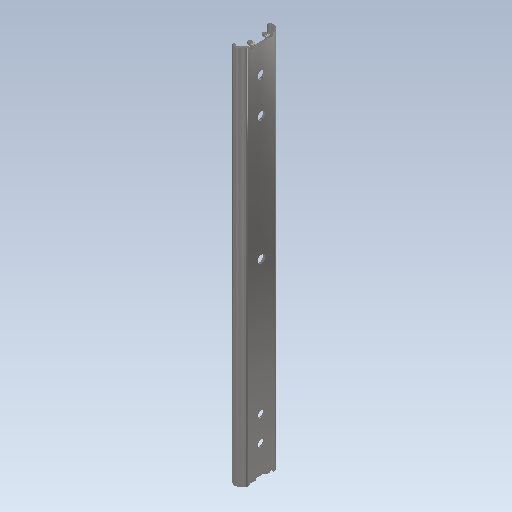
# Autodesk Inventor part: SSRC215_or
Saved by Autodesk Inventor 2021.2 (Build 252289000, 289)
## iProperties
Part Number: SSRC215_or
Material: ステンレス鋼
Catalog Web Link: www.cadenas.de
Description: SSRC2_outer_rail-Slide Rails - Load Rating: 137N ~ 177N/2 pcs - Light Load / Compact - Stainless Steel - Tow-Step
Vendor: MISUMI
Document SubType Name: Modeling
Designer: partserver
Manufacturer: MISUMI
Mass: 19.4626 g
Surface Area: 63.9405 cm^2
Volume: 2.43283 cm^3
Density: 8 g/cm^3
Appearance: 半つや出し
Category: PARTsolutions
Company: MISUMI
PSOL_IDENT_0: {$CADENAS_DATA\23d-libs\misumi\metric\07_slide_rails\ssrc2\ssrc2_outer_rail.prj},167 {VTYP=3D},{NB=S
PSOL_IDENT_1: SRC215_or},{LINA=SSRC215},{NN=SSRC2_outer_rail},{DATE=30.03.2018 01:39:53},{GEOMDATE=30.06.2015 02:0
PSOL_IDENT_2: 1:15},{VERSION=},{LINEID=30},{WBVAR=},{WBNUMERIC=}  {NB=SSRC215_or},{LINA=SSRC215},{KT=DUMMY},{PN=SS
PSOL_IDENT_3: RC215},{TYPE=SSRC2},{NO=15},{L=150},{S=94.5},{A=63},{B=126},{C=63},{D=126},{E=102},{F=98}
NB: SSRC215_or
NN: SSRC2_outer_rail
NT: Slide Rails - Load Rating: 137N ~ 177N/2 pcs - Light Load / Compact - Stainless Steel - Tow-Step
NBSYN: $PN._or
LINA: SSRC215
CATALOG: Misumi
PN: SSRC215
NO: 15
L: 150
S: 94.5
A: 63
B: 126
C: 63
D: 126
E: 102
F: 98
SUPPLIER: MISUMI
ARTICLENO: SSRC215_or
BOMINFO: SSRC215
CREATOR: CADENAS GmbH
Title: SSRC215
Author: Cadenas PARTsolutions
Comments: Slide Rails - Load Rating: 137N ~ 177N/2 pcs - Light Load / Compact - Stainless Steel - Tow-Step
Autodesk Inventor part; units mm, degrees
sketch "_____1" plane through (0, 0, 0) normal (0, 0, 1) x (1, 0, 0)
  line L0 (-2.85, 5.26) -> (-2.85, -5.26)
  arc A0 (-2.85, -5.26) -> (-2.0307, -6.4679) centre (-1.55, -5.26) ccw
  line L1 (-2.0307, -6.4679) -> (-1.8349, -6.5458)
  arc A1 (-1.8349, -6.5458) -> (1.43, -7.1482) centre (0, -5.75) ccw
  line L2 (1.43, -7.1482) -> (1.43, -6.5756)
  line L3 (1.43, -6.5756) -> (1.0392, -6.35)
  arc A2 (-1.1009, -6.2275) -> (1.0392, -6.35) centre (0, -5.75) ccw
  arc A3 (-1.1009, -6.2275) -> (-1.5391, -5.8025) centre (-1.8349, -6.5458) ccw
  line L4 (-1.5391, -5.8025) -> (-1.7349, -5.7246)
  arc A4 (-2.05, -5.26) -> (-1.7349, -5.7246) centre (-1.55, -5.26) ccw
  line L5 (-2.05, -5.26) -> (-2.05, 5.26)
  arc A5 (-1.7349, 5.7246) -> (-2.05, 5.26) centre (-1.55, 5.26) ccw
  line L6 (-1.7349, 5.7246) -> (-1.5391, 5.8025)
  arc A6 (-1.5391, 5.8025) -> (-1.1009, 6.2275) centre (-1.8349, 6.5458) ccw
  arc A7 (1.0392, 6.35) -> (-1.1009, 6.2275) centre (0, 5.75) ccw
  line L7 (1.0392, 6.35) -> (1.43, 6.5756)
  line L8 (1.43, 6.5756) -> (1.43, 7.1482)
  arc A8 (1.43, 7.1482) -> (-1.8349, 6.5458) centre (0, 5.75) ccw
  line L9 (-1.8349, 6.5458) -> (-2.0307, 6.4679)
  arc A9 (-2.0307, 6.4679) -> (-2.85, 5.26) centre (-1.55, 5.26) ccw
  constraints: 20 end point, 20 point on circle, 10 centre point
extrude "Extrusion1" add sketch "_____1" against normal blind 150
sketch "_____3" plane through (0, 0, 0) normal (0, 0, 1) x (1, 0, 0)
  line L0 (-2.05, 3.6) -> (-2.05, 2.2)
  line L1 (-2.05, 2.2) -> (-0.95, 2.2)
  arc A0 (-0.95, 2.2) -> (-0.45, 2.7) centre (-0.95, 2.7) ccw
  line L2 (-0.45, 2.7) -> (-0.45, 2.9484)
  arc A1 (-0.45, 2.9484) -> (-0.8206, 3.4314) centre (-0.95, 2.9484) ccw
  line L3 (-0.8206, 3.4314) -> (-1.45, 3.6)
  line L4 (-1.45, 3.6) -> (-2.05, 3.6)
  constraints: 10 end point, 4 point on circle, 2 centre point
extrude "Extrusion2" add sketch "_____3" against normal blind 0.8
sketch "_____5" plane through (0, 0, 0) normal (0, 0, 1) x (1, 0, 0)
  line L0 (-2.05, -3.6) -> (-1.45, -3.6)
  line L1 (-1.45, -3.6) -> (-0.8206, -3.4314)
  arc A0 (-0.8206, -3.4314) -> (-0.45, -2.9484) centre (-0.95, -2.9484) ccw
  line L2 (-0.45, -2.9484) -> (-0.45, -2.7)
  arc A1 (-0.45, -2.7) -> (-0.95, -2.2) centre (-0.95, -2.7) ccw
  line L3 (-0.95, -2.2) -> (-2.05, -2.2)
  line L4 (-2.05, -2.2) -> (-2.05, -3.6)
  constraints: 10 end point, 4 point on circle, 2 centre point
extrude "Extrusion3" add sketch "_____5" against normal blind 0.8
sketch "_____4" plane through (0, 0, 0) normal (1, 0, 0) x (0, 1, 0)
  line L0 (7.75, 1) -> (-7.75, 1)
  line L1 (-7.75, 1) -> (-7.75, 0)
  line L2 (-7.75, 0) -> (-4.9, 0)
  arc A0 (-4.6, -0.3) -> (-4.9, 0) centre (-4.9, -0.3) ccw
  line L3 (-4.6, -0.3) -> (-4.6, -0.7)
  arc A1 (-4.6, -0.7) -> (-4.1, -1.2) centre (-4.1, -0.7) ccw
  arc A2 (-4.1, -1.2) -> (-3.6, -0.7) centre (-4.1, -0.7) ccw
  line L4 (-3.6, -0.7) -> (-3.6, 0)
  line L5 (-3.6, 0) -> (-2.2, 0)
  line L6 (-2.2, 0) -> (-2.2, -0.7)
  arc A3 (-2.2, -0.7) -> (-1.7, -1.2) centre (-1.7, -0.7) ccw
  line L7 (-1.7, -1.2) -> (1.7, -1.2)
  arc A4 (1.7, -1.2) -> (2.2, -0.7) centre (1.7, -0.7) ccw
  line L8 (2.2, -0.7) -> (2.2, 0)
  line L9 (2.2, 0) -> (3.6, 0)
  line L10 (3.6, 0) -> (3.6, -0.7)
  arc A5 (3.6, -0.7) -> (4.1, -1.2) centre (4.1, -0.7) ccw
  arc A6 (4.1, -1.2) -> (4.6, -0.7) centre (4.1, -0.7) ccw
  line L11 (4.6, -0.7) -> (4.6, -0.3)
  arc A7 (4.9, 0) -> (4.6, -0.3) centre (4.9, -0.3) ccw
  line L12 (4.9, 0) -> (7.75, 0)
  line L13 (7.75, 0) -> (7.75, 1)
  constraints: 28 end point, 16 point on circle, 8 centre point
extrude "Extrusion4" cut sketch "_____4" against normal blind 4.28
sketch "_____6" plane through (0, 0, 0) normal (0, 1, 0) x (1, 0, 0)
  line L0 (-2.85, 0.8) -> (-2.85, 0)
  line L1 (-2.85, 0) -> (-2.05, 0)
  arc A0 (-2.85, 0.8) -> (-2.05, 0) centre (-2.05, 0.8) ccw
  constraints: 4 end point, 2 point on circle, 1 centre point
extrude "Extrusion5" cut sketch "_____6" along normal mid plane 8.2
sketch "_____2" plane through (0, 0, -150) normal (0, 0, 1) x (1, 0, 0)
  line L0 (-2.05, 3.6) -> (-2.05, 2.2)
  line L1 (-2.05, 2.2) -> (-0.95, 2.2)
  arc A0 (-0.95, 2.2) -> (-0.45, 2.7) centre (-0.95, 2.7) ccw
  line L2 (-0.45, 2.7) -> (-0.45, 2.9484)
  arc A1 (-0.45, 2.9484) -> (-0.8206, 3.4314) centre (-0.95, 2.9484) ccw
  line L3 (-0.8206, 3.4314) -> (-1.45, 3.6)
  line L4 (-1.45, 3.6) -> (-2.05, 3.6)
  constraints: 10 end point, 4 point on circle, 2 centre point
extrude "Extrusion6" add sketch "_____2" along normal blind 0.8
sketch "_____7" plane through (0, 0, -150) normal (0, 0, 1) x (1, 0, 0)
  line L0 (-2.05, -3.6) -> (-1.45, -3.6)
  line L1 (-1.45, -3.6) -> (-0.8206, -3.4314)
  arc A0 (-0.8206, -3.4314) -> (-0.45, -2.9484) centre (-0.95, -2.9484) ccw
  line L2 (-0.45, -2.9484) -> (-0.45, -2.7)
  arc A1 (-0.45, -2.7) -> (-0.95, -2.2) centre (-0.95, -2.7) ccw
  line L3 (-0.95, -2.2) -> (-2.05, -2.2)
  line L4 (-2.05, -2.2) -> (-2.05, -3.6)
  constraints: 10 end point, 4 point on circle, 2 centre point
extrude "Extrusion7" add sketch "_____7" along normal blind 0.8
sketch "_____8" plane through (-2.85, 0, 0) normal (1, 0, 0) x (0, 0, -1)
  arc A0 (148.8, -4.1) -> (149.3, -4.6) centre (149.3, -4.1) ccw
  line L0 (149.3, -4.6) -> (149.7, -4.6)
  arc A1 (150, -4.9) -> (149.7, -4.6) centre (149.7, -4.9) ccw
  line L1 (150, -4.9) -> (150, -7.75)
  line L2 (150, -7.75) -> (151, -7.75)
  line L3 (151, -7.75) -> (151, 7.75)
  line L4 (151, 7.75) -> (150, 7.75)
  line L5 (150, 7.75) -> (150, 4.9)
  arc A2 (149.7, 4.6) -> (150, 4.9) centre (149.7, 4.9) ccw
  line L6 (149.7, 4.6) -> (149.3, 4.6)
  arc A3 (149.3, 4.6) -> (148.8, 4.1) centre (149.3, 4.1) ccw
  arc A4 (148.8, 4.1) -> (149.3, 3.6) centre (149.3, 4.1) ccw
  line L7 (149.3, 3.6) -> (150, 3.6)
  line L8 (150, 3.6) -> (150, 2.2)
  line L9 (150, 2.2) -> (149.3, 2.2)
  arc A5 (149.3, 2.2) -> (148.8, 1.7) centre (149.3, 1.7) ccw
  line L10 (148.8, 1.7) -> (148.8, -1.7)
  arc A6 (148.8, -1.7) -> (149.3, -2.2) centre (149.3, -1.7) ccw
  line L11 (149.3, -2.2) -> (150, -2.2)
  line L12 (150, -2.2) -> (150, -3.6)
  line L13 (150, -3.6) -> (149.3, -3.6)
  arc A7 (149.3, -3.6) -> (148.8, -4.1) centre (149.3, -4.1) ccw
  constraints: 28 end point, 16 point on circle, 8 centre point
extrude "Extrusion8" cut sketch "_____8" along normal blind 0.8
sketch "_____9" plane through (0, 0, 0) normal (0, 1, 0) x (1, 0, 0)
  arc A0 (-2.05, 150) -> (-2.85, 149.2) centre (-2.05, 149.2) ccw
  line L0 (-2.05, 150) -> (-2.85, 150)
  line L1 (-2.85, 150) -> (-2.85, 149.2)
  constraints: 4 end point, 2 point on circle, 1 centre point
extrude "Extrusion9" cut sketch "_____9" along normal mid plane 8.2
sketch "Sketch10" plane through (-2.05, 5.26, 0) normal (1, 0, 0) x (0, 0, -1)
  point P0 (12, -5.26)
hole "Hole1" at (-2.05, 0, -12) direction (-1, 0, 0) diameter 2.8 depth 0.8
pattern_linear "Rectangular Pattern1" count 2 spacing 10 along (0, 0, -1) of "Hole1"
sketch "_____12" plane through (-2.85, 0, 0) normal (1, 0, 0) x (0, 0, -1)
  arc A0 (123.8, 1.4) -> (123.8, -1.4) centre (123.8, 0) ccw
  line L0 (123.8, -1.4) -> (124.2, -1.4)
  arc A1 (124.2, -1.4) -> (124.2, 1.4) centre (124.2, 0) ccw
  line L1 (124.2, 1.4) -> (123.8, 1.4)
  constraints: 4 end point, 4 point on circle, 2 centre point
extrude "Extrusion10" cut sketch "_____12" along normal blind 0.8
sketch "_____13" plane through (-2.85, 0, 0) normal (1, 0, 0) x (0, 0, -1)
  arc A0 (137.8, 1.4) -> (137.8, -1.4) centre (137.8, 0) ccw
  line L0 (137.8, -1.4) -> (138.2, -1.4)
  arc A1 (138.2, -1.4) -> (138.2, 1.4) centre (138.2, 0) ccw
  line L1 (138.2, 1.4) -> (137.8, 1.4)
  constraints: 4 end point, 4 point on circle, 2 centre point
extrude "Extrusion11" cut sketch "_____13" along normal blind 0.8
sketch "_____14" plane through (-2.85, 0, 0) normal (1, 0, 0) x (0, 0, -1)
  arc A0 (74.8, 1.4) -> (74.8, -1.4) centre (74.8, 0) ccw
  line L0 (74.8, -1.4) -> (75.2, -1.4)
  arc A1 (75.2, -1.4) -> (75.2, 1.4) centre (75.2, 0) ccw
  line L1 (75.2, 1.4) -> (74.8, 1.4)
  constraints: 4 end point, 4 point on circle, 2 centre point
extrude "Extrusion12" cut sketch "_____14" along normal blind 0.8
ref_plane "to_retainer_XY" through (0, 0, 0) normal (0, 0, 1) x (1, 0, 0)
ref_plane "to_retainer_YZ" through (0, 0, 0) normal (1, 0, 0) x (0, 1, 0)
ref_plane "to_retainer_ZX" through (0, 0, 0) normal (0, 1, 0) x (0, 0, 1)
body "Solid1"
